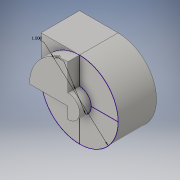
# Autodesk Inventor part: dope
Saved by Autodesk Inventor 2016 (Build 200138000, 138)
## iProperties
Created: 2018-02-12
Part Number: dope
Material: Generic
Document SubType Name: Modeling
Designer: sun01147
Density: 1 g/cm^3
Appearance: Default
Author: sun01147
Autodesk Inventor part; units mm, degrees
ref_plane "YZ Plane" through (0, 0, 0) normal (1, 0, 0) x (0, 1, 0)
ref_plane "XZ Plane" through (0, 0, 0) normal (0, 1, 0) x (-1, 0, 0)
ref_plane "XY Plane" through (0, 0, 0) normal (0, 0, 1) x (1, 0, 0)
sketch "Sketch1" plane through (0, 0, 0) normal (0, 0, 1) x (1, 0, 0)
  circle A0 centre (0, 0) radius 12.7
  circle A1 centre (0, 0) radius 3.81
  line L0 (0, 12.7) -> (0, 0)
  line L1 (0, 0) -> (12.7, 0)
  line L2 (0, -12.7) -> (0, 0)
  line L3 (-12.7, 0) -> (0, 0)
  line L4 (0, 3.81) -> (0, 0)
  line L5 (3.81, 0) -> (0, 0)
  line L6 (0, -3.81) -> (0, 0)
  line L7 (-3.81, 0) -> (0, 0)
  dimension "d0" = 25.4
  dimension "d1" = 7.62
  constraints: 16 end point, 8 point on circle, 6 point on line, 4 perpendicular, 3 collinear, 2 centre point, 2 coincident, 1 vertical
  measures "d0" diameter of A0
  measures "d1" diameter of A1
extrude "Extrusion1" add sketch "Sketch1" against normal blind 12.7 contours L1 A1 L0 A0 | A0 L2 A1 L1 | L0 A1 L3 A0 | A0 L3 A1 L2
extrude "Extrusion2" cut sketch "Sketch1" against normal blind 12.7 contours L0 A1 L3 A0 | L0 L3 A1
sketch "Sketch2" plane through (0, 3.81, 0) normal (-1, 0, 0) x (0, 0, 1)
  line L0 (-12.7, 8.89) -> (-12.7, -16.51) projected
  line L1 (0, 0) -> (-12.7, 0) projected
  line L2 (-12.7, 8.89) -> (-12.7, 0)
  line L3 (-12.7, 0) -> (0, 0)
  line L4 (0, 8.89) -> (0, -16.51) projected
  line L5 (0, 0) -> (0, 8.89)
  line L6 (-12.7, 8.89) -> (0, 8.89) projected
  line L7 (0, 8.89) -> (-12.7, 8.89)
  point P0 (0, -3.81)
  point P1 (-12.7, -3.81)
  constraints: 8 end point, 4 collinear
extrude "Extrusion3" add sketch "Sketch2" along normal blind 12.7
extrude "Extrusion4" add sketch "Sketch1" along normal blind 3.81 contours A1 L2 L1 | L0 L3 A1
extrude "Extrusion5" add sketch "Sketch1" along normal blind 3.81 contours L1 L0 A1
extrude "Extrusion6" add sketch "Sketch1" along normal blind 3.81 contours L0 A1 L3 A0
body "Solid1"
